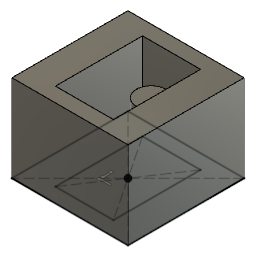
complex_object (Autodesk Fusion 360 design; units mm, degrees)
Autodesk Fusion 360 part; units mm, degrees
sketch "Sketch1" plane through (0, 0, 0) normal (0, 1, 0) x (1, 0, 0)
  line L0 (1000, 1000) -> (-1000, 1000)
  line L1 (-1000, 1000) -> (-1000, -1000)
  line L2 (-1000, -1000) -> (1000, -1000)
  line L3 (1000, -1000) -> (1000, 1000)
  line L4 (1000, 1000) -> (-1000, -1000) construction
  line L5 (-1000, 1000) -> (1000, -1000) construction
  line L6 (500, 750) -> (-500, 750)
  line L7 (-500, 750) -> (-500, -750)
  line L8 (-500, -750) -> (500, -750)
  line L9 (500, -750) -> (500, 750)
  line L10 (500, 750) -> (-500, -750) construction
  line L11 (-500, 750) -> (500, -750) construction
  constraint horizontal L0
  constraint perpendicular L0 L1
  constraint parallel L0 L2
  constraint parallel L1 L3
  constraint coincident L4 origin
  constraint coincident L5 origin
  constraint horizontal L6
  constraint perpendicular L6 L7
  constraint parallel L6 L8
  constraint parallel L7 L9
  constraint coincident L10 origin
  constraint coincident L11 origin
extrude "Extrude1" add sketch "Sketch1" along normal blind 100 contours L0 L1 L2 L3 | L6 L7 L8 L9 makes body 1
extrude "Extrude2" add sketch "Sketch1" along normal blind 1500 bodies 1
sketch "Sketch2" plane through (0, 0, 0) normal (1, 0, 0) x (0, 0, -1)
ref_plane "WorkPlane1" through (0, 1000, 0) normal (0, 1, 0) x (0, 0, 1)
cylinder "CylinderPrimitive1" add diameter 510 height -500 placed x (1, 0, 0) y (0, 0, -1) z (0, 1, 0) at (0, 1000, 0) separate body makes body 2
chamfer "Chamfer1" distance 200 angle 45 1 edges at (-92.2119, 500, 237.7435) on bodies 2
move_body "Move1" bodies 2 to x (1, 0, 0) y (0, 1, 0) z (0, 0, 1) at (0, 0, -400)
sphere "SpherePrimitive1" add diameter 500 placed x (1, 0, 0) y (0, 0, -1) z (0, 1, 0) at (0, 1000, 0) separate body makes body 3
move_body "MoveFace1" bodies 3 to x (1, 0, 0) y (0, 1, 0) z (0, 0, 1) at (0, 0, 400) on bodies 3
move_body "MoveFace2" bodies 3 to x (1, 0, 0) y (0, 1, 0) z (0, 0, 1) at (0, -300, 0) on bodies 3
